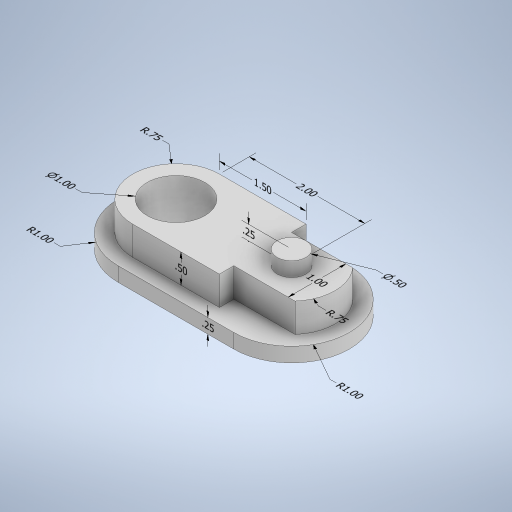
# Autodesk Inventor part: Part4
Saved by Autodesk Inventor 2023 (Build 270158000, 158)
## iProperties
Created: 2023-07-11
Part Number: Part4
Material: Generic
Document SubType Name: Modeling
Designer: Greg
Density: 1 g/cm^3
Appearance: Default
Author: Greg
Autodesk Inventor part; units mm, degrees
ref_plane "YZ Plane" through (0, 0, 0) normal (1, 0, 0) x (0, 1, 0)
ref_plane "XZ Plane" through (0, 0, 0) normal (0, 1, 0) x (-1, 0, 0)
ref_plane "XY Plane" through (0, 0, 0) normal (0, 0, 1) x (1, 0, 0)
sketch "Sketch1" plane through (0, 0, 0) normal (0, 1, 0) x (-1, 0, 0)
  arc A0 (0, -25.4) -> (0, 25.4) centre (0, 0) ccw
  arc A1 (-50.8, 25.4) -> (-50.8, -25.4) centre (-50.8, 0) ccw
  line L0 (0, 25.4) -> (-50.8, 25.4)
  line L1 (0, -25.4) -> (-50.8, -25.4)
  dimension "d0" = 50.8
  constraints: 4 end point, 4 point on circle, 2 centre point, 2 tangent, 1 coincident
  measures "d0" diameter of A0
extrude "Extrusion1" add sketch "Sketch1" along normal blind 6.35
sketch "Sketch2" plane through (0, 6.35, 0) normal (0, 1, 0) x (1, 0, 0)
  arc A0 (0, 19.05) -> (0, -19.05) centre (0, 0) ccw
  line L0 (0, 19.05) -> (38.1, 19.05)
  line L1 (0, -19.05) -> (38.1, -19.05)
  arc A1 (50.8, -25.4) -> (50.8, 25.4) centre (50.8, 0) ccw projected
  arc A2 (64.999, -12.7) -> (64.999, 12.7) centre (50.8, 0) ccw
  line L2 (50.8, 12.7) -> (64.999, 12.7)
  line L3 (50.8, -12.7) -> (64.999, -12.7)
  line L4 (50.8, -12.7) -> (38.1, -12.7)
  line L5 (50.8, 12.7) -> (38.1, 12.7)
  line L6 (38.1, 19.05) -> (38.1, 12.7)
  line L7 (38.1, -19.05) -> (38.1, -12.7)
  dimension "d6" = 38.1
  dimension "d7" = 38.1
  constraints: 16 end point, 6 horizontal, 4 point on circle, 2 centre point, 2 coincident, 2 perpendicular, 2 tangent
  measures "d6" distance of L0.start L0.end
  measures "d7" distance of L1.start L1.end
extrude "Extrusion2" add sketch "Sketch2" along normal blind 12.7
sketch "Sketch3" plane through (0, 19.05, 0) normal (0, 1, 0) x (1, 0, 0)
  circle A0 centre (0, 0) radius 12.7
  dimension "d13" = 25.4
  constraints: 1 centre point, 1 coincident
  measures "d13" diameter of A0
extrude "Extrusion3" cut sketch "Sketch3" against normal blind 25.4
sketch "Sketch4" plane through (0, 19.05, 0) normal (0, 1, 0) x (1, 0, 0)
  arc A0 (64.999, -12.7) -> (64.999, 12.7) centre (50.8, 0) ccw projected
  circle A1 centre (50.8, 0) radius 6.35
  point P0 (0, 0)
  dimension "d16" = 12.7
  constraints: 1 centre point, 1 coincident
  measures "d16" diameter of A1
extrude "Extrusion4" add sketch "Sketch4" along normal blind 6.35
body "Solid1"
